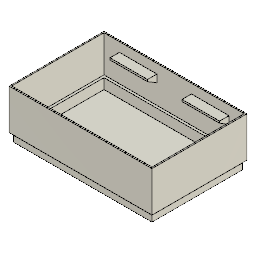
Component Storage (Autodesk Fusion 360 design; units mm, degrees)
Autodesk Fusion 360 part; units mm, degrees
sketch "Sketch1" plane through (0, 0, 0) normal (0, 0, 1) x (1, 0, 0)
  line L0 (38.4375, -25.625) -> (-38.4375, -25.625)
  line L1 (-38.4375, -25.625) -> (-38.4375, 25.625)
  line L2 (-38.4375, 25.625) -> (38.4375, 25.625)
  line L3 (38.4375, 25.625) -> (38.4375, -25.625)
  line L4 (38.4375, -25.625) -> (-38.4375, 25.625) construction
  line L5 (-38.4375, -25.625) -> (38.4375, 25.625) construction
  line L6 (37.4375, -24.625) -> (-37.4375, -24.625)
  line L7 (-37.4375, -24.625) -> (-37.4375, 24.625)
  line L8 (-37.4375, 24.625) -> (37.4375, 24.625)
  line L9 (37.4375, 24.625) -> (37.4375, -24.625)
  line L10 (-36.1518, -23.3393) -> (-36.1518, 23.3393)
  line L11 (-36.1518, 23.3393) -> (36.1518, 23.3393)
  line L12 (36.1518, 23.3393) -> (36.1518, -23.3393)
  line L13 (36.1518, -23.3393) -> (-36.1518, -23.3393)
  line L14 (38.1518, -25.3393) -> (-38.1518, -25.3393)
  line L15 (-38.1518, -25.3393) -> (-38.1518, 25.3393)
  line L16 (-38.1518, 25.3393) -> (38.1518, 25.3393)
  line L17 (38.1518, 25.3393) -> (38.1518, -25.3393)
  line L18 (36.9375, -24.125) -> (-36.9375, -24.125)
  line L19 (-36.9375, -24.125) -> (-36.9375, 24.125)
  line L20 (-36.9375, 24.125) -> (36.9375, 24.125)
  line L21 (36.9375, 24.125) -> (36.9375, -24.125)
  dimension "d7" = 76.875
  dimension "d8" = 51.25
  dimension "d10" = 1
  dimension "d18" = 2.2857
  dimension "d34" = 0.2857
  dimension "d36" = 1.5
  constraint horizontal L0
  constraint perpendicular L0 L1
  constraint parallel L0 L2
  constraint parallel L1 L3
  constraint coincident L4 origin
  constraint coincident L5 origin
  measures "d7" distance of L1.end L2.end
  measures "d8" distance of L0.end L1.end
extrude "Extrude1" add sketch "Sketch1" along normal blind 26 contours L0 L1 L2 L3 | L14 L15 L16 L17
extrude "Extrude7" cut sketch "Sketch1" along normal through all contours L0 L1 L2 L3
extrude "Extrude2" add sketch "Sketch1" along normal blind 1 contours L6 L7 L8 L9 | L10 L11 L12 L13 | L18 L19 L20 L21
extrude "Extrude4" add sketch "Sketch1" along normal blind 6.5 contours L6 L7 L8 L9 | L18 L19 L20 L21
extrude "Extrude5" cut sketch "Sketch1" along normal blind 4.5 contours L0 L1 L2 L3 | L14 L15 L16 L17
extrude "Extrude8" cut sketch "Sketch1" along normal up to surface (4.5 mm away) contours L6 L7 L8 L9
sketch "Sketch2" plane through (0, 24.625, 0) normal (0, -1, 0) x (1, 0, 0)
  line L0 (-37.4375, 6.5) -> (37.4375, 6.5)
  line L1 (37.4375, 6.5) -> (37.4375, 26)
  line L2 (37.4375, 26) -> (-37.4375, 26)
  line L3 (-37.4375, 26) -> (-37.4375, 6.5)
  line L4 (-29.2187, 21) -> (-9.2187, 21)
  line L5 (-9.2187, 21) -> (-9.2187, 20)
  line L6 (-9.2187, 20) -> (-29.2187, 20)
  line L7 (-29.2187, 20) -> (-29.2187, 21)
  line L8 (-19.2187, 26) -> (-19.2187, 21) construction
  point P0 (-19.2187, 21)
  point P1 (-19.2187, 21)
  point P2 (-38.1518, 26)
  point P3 (-38.4375, 0)
  dimension "d26" = 20
  dimension "d27" = 1
  dimension "d30" = 5
  dimension "d64" = 19.2188
  constraint horizontal L4
  constraint vertical L5
  constraint horizontal L6
  constraint vertical L7
  constraint midpoint L4 P1
  constraint coincident P1 P0
  constraint perpendicular L2 L8
  constraint coincident L2 L8.start
  measures "d26" distance of L4.start L4.end
  measures "d27" distance of L4.start L6.end
  measures "d30" distance of L8.start P1
  measures "d64" horizontal distance of L8.start P3
extrude "Extrude6" add sketch "Sketch2" along normal blind 5 contours L4 L5 L6 L7
sketch "Sketch3" plane through (-9.2187, 0, 0) normal (1, 0, 0) x (0, 1, 0)
  line L0 (24.625, 20) -> (24.625, 21)
  line L1 (24.625, 21) -> (19.625, 21)
  line L2 (19.625, 21) -> (19.625, 20)
  line L3 (19.625, 20) -> (24.625, 20)
  line L4 (19.625, 20) -> (24.625, 20)
  line L5 (24.625, 17) -> (19.625, 20)
  line L6 (24.625, 20) -> (24.625, 17)
  dimension "d46" = 3
  constraint coincident L2.end L3.start
  constraint coincident L0.start L3.end
  constraint vertical L0.start L5.start
  measures "d46" distance of L0.start L5.start
extrude "Extrude9" add sketch "Sketch3" against normal blind 1 contours L3 L4 L5 L6
ref_plane "WorkPlane1" through (-19.2187, 22.125, 19) normal (1, 0, 0) x (0, 0, 1)
mirror "Mirror1" about plane through (-19.2187, 22.125, 19) normal (1, 0, 0) of "Extrude9"
pattern_linear "R-Pattern1" count 2 spacing 38.4375 along (1, 0, 0) of "Extrude6", "Extrude9", "Mirror1"
ref_plane "WorkPlane2" through (0, 0, 16.25) normal (0, 1, 0) x (-1, 0, 0)
mirror "Mirror2" about plane through (0, 0, 16.25) normal (0, 1, 0) of "Extrude6", "Extrude9", "Mirror1", "R-Pattern1"
chamfer "Chamfer1" [suppressed]
chamfer "Chamfer3" [suppressed]
equation "boxiw = 205 mm" comment "Internal width of larger container"
equation "boxil = 205 mm" comment "Internal length of larger container"
equation "cupnumw = 8 / 3" comment "Number of cups along the width of the box"
equation "cupw = boxiw / cupnumw"
equation "cupl = boxil / cupnuml"
equation "cupnuml = 8 / 2" comment "Number of cups along the length of the box"
equation "d7 = cupw"
equation "d8 = cupl"
equation "thick = 1 mm" comment "Thickness of the cups' parts"
equation "d10 = thick"
equation "boxih = 68 mm" comment "Internal height of larger container"
equation "cupnumh = 6 / 2" comment "Number of cups along the height of the box"
equation "cuph = ( boxih + overlap * ( cupnumh - 1 ) ) / cupnumh"
equation "d14 = cuph"
equation "d16 = thick"
equation "d18 = d10 * 2 + d34"
equation "overlap = 5 mm"
equation "d22 = overlap + thick + tol"
equation "d24 = overlap - tol"
equation "d27 = thick"
equation "d30 = overlap"
equation "tol = 0.5 mm"
equation "d34 = tol / 1.75"
equation "d36 = d10 + tol"
equation "d47 = -thick"
equation "d55 = tol"
equation "handlenum = floor(cupw / 30 mm)"
equation "handlespace = cupw / ( handlenum )"
equation "d59 = handlenum"
equation "d61 = -handlespace"
equation "d64 = handlespace / 2"
named bodies: "cup"
